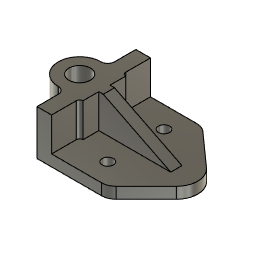
H2-A3 (Autodesk Fusion 360 design; units mm, degrees)
Autodesk Fusion 360 part; units mm, degrees
sketch "Sketch1" plane through (0, 0, 0) normal (0, 0, 1) x (1, 0, 0)
  line L0 (16.3701, -44) -> (-33.5, -44)
  line L1 (-33.5, 44) -> (12.6952, 44)
  line L2 (-26.5, 5) -> (-30.5, 5) construction
  line L3 (-30.5, -5) -> (-26.5, -5) construction
  circle A0 centre (-2.5, 25) radius 5
  circle A1 centre (-2.5, -25) radius 5
  line L4 (46.935, 13.435) -> (46.9571, 13.4571)
  line L5 (46.935, -13.435) -> (16.3701, -44)
  line L6 (46.9571, 13.4571) -> (12.6952, 44)
  line L7 (-33.5, 44) -> (-46.5, 44)
  line L8 (-46.5, -44) -> (-33.5, -44)
  circle A2 centre (-52.5, 0) radius 9.5
  arc A3 (-52.5, 19) -> (-46.5, 25) centre (-52.5, 25) ccw
  arc A4 (-46.5, -25) -> (-52.5, -19) centre (-52.5, -25) ccw
  line L9 (-46.5, 25) -> (-46.5, 44) construction
  line L10 (-46.5, 44) -> (-46.5, 25)
  arc A5 (-52.5, 19) -> (-52.5, -19) centre (-52.5, 0) ccw
  line L11 (-46.5, -44) -> (-46.5, -25) construction
  line L12 (-46.5, -25) -> (-46.5, -44)
  line L13 (-33.5, -44) -> (-26.5, -44) construction
  arc A6 (-30.5, -19) -> (-33.5, -22) centre (-30.5, -22) ccw
  arc A7 (-33.5, 22) -> (-30.5, 19) centre (-30.5, 22) ccw
  line L14 (-33.5, -22) -> (-33.5, -44) construction
  line L15 (-33.5, 44) -> (-33.5, 22) construction
  line L16 (-33.5, 22) -> (-33.5, 44)
  line L17 (-33.5, 22) -> (-33.5, 44)
  line L18 (-33.5, -44) -> (-33.5, -22)
  line L19 (-33.5, -44) -> (-33.5, -22)
  arc A8 (46.935, -13.435) -> (46.1432, 14.1827) centre (33.5, 0) ccw
  line L20 (-30.5, -19) -> (-30.5, -5)
  line L21 (-30.5, 5) -> (-30.5, 19)
  line L22 (-30.5, -5) -> (-26.5, -5)
  line L23 (-26.5, -5) -> (-26.5, 5)
  line L24 (-26.5, 5) -> (-30.5, 5)
  dimension "d2" = 88
  dimension "d4" = 10
  dimension "d5" = 39
  dimension "d8" = 10
  dimension "d9" = 10
  dimension "d10" = 38
  dimension "d13" = 13
  dimension "d17" = 19
  dimension "d18" = 38
  dimension "d20" = 12
  dimension "d21" = 12
  dimension "d22" = 7
  dimension "d25" = 6
  dimension "d26" = 6
  dimension "d27" = 4
  constraint horizontal L0
  constraint perpendicular L0 L19
  constraint parallel L0 L1
  constraint perpendicular L2 L19
  constraint tangent L5 A8
  constraint tangent L6 A8
  constraint coincident L4.start A8
  constraint horizontal L7
  constraint vertical L10
  constraint horizontal L8
  constraint vertical L18
  constraint vertical L11
  constraint concentric A2 A5
  constraint tangent A4 L10
  constraint coincident A4.start L10
  constraint collinear L9 L11
  constraint horizontal L13
  constraint vertical L15
  constraint tangent A6 L15
  constraint tangent A7 L18
  constraint coincident A7.start L19
  constraint collinear L14 L15
  constraint collinear L16 L19
  constraint collinear L17 L18
  constraint coincident L6 A8.end
  constraint perpendicular L3 L20
  constraint perpendicular L2 L21
  constraint perpendicular L20 L22
  constraint perpendicular L2 L23
  measures "d2" distance of L0.end L1.start
  measures "d4" distance of L2 L3
  measures "d5" distance of L0 L3
  measures "d8" diameter of A0
  measures "d9" diameter of A1
  measures "d10" diameter of A8
  measures "d13" distance of L1.start L7.end
  measures "d17" diameter of A2
  measures "d18" diameter of A5
  measures "d20" diameter of A4
  measures "d21" diameter of A3
  measures "d22" distance of L0.end L13.end
  measures "d25" diameter of A6
  measures "d26" diameter of A7
  measures "d27" distance of L3.start L3.end
extrude "Extrude1" add sketch "Sketch1" along normal blind 40 contours L7 L8 A3 A4 L10 A5 L12 A6 A7 L16 L17 L18 L19 L20 L21 L22 L23 L24
extrude "Extrude2" add sketch "Sketch1" along normal blind 10 contours L0 L1 L5 L6 A6 A7 L16 L17 L18 L19 A8 L20 L21 L22 L23 L24
sketch "Sketch2" plane through (0, 0, 0) normal (0, 1, 0) x (1, 0, 0)
  line L0 (-26.5, -40) -> (-26.5, -10)
  line L1 (-26.5, -10) -> (33.5, -10)
  line L2 (33.5, -10) -> (-26.5, -40)
  dimension "d32" = 60
  constraint vertical L0
  constraint perpendicular L0 L1
  measures "d32" distance of L0.end L1.end
extrude "Extrude3" add sketch "Sketch2" along normal mid plane 10
fillet "Fillet1" radius 13 1 edges at (16.3701, -44, 5)
fillet "Fillet2" radius 13 1 edges at (12.6952, 44, 5)
equation "d5 = ( ( 88 - 10 ) / 2 ) * 1 mm"
equation "d10 = ( 19 * 2 ) * 1 mm"
